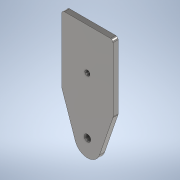
# Autodesk Inventor part: Frame2
Saved by Autodesk Inventor 2020 (Build 240168000, 168)
## iProperties
Created: 2022-06-23
Part Number: Frame2
Material: Steel, Carbon
Document SubType Name: Modeling
Designer: karimi2
Density: 7.85 g/cm^3
Appearance: Semi-Polished
Author: karimi2
Autodesk Inventor part; units mm, degrees
ref_plane "YZ Plane" through (0, 0, 0) normal (1, 0, 0) x (0, 1, 0)
ref_plane "XZ Plane" through (0, 0, 0) normal (0, 1, 0) x (-1, 0, 0)
ref_plane "XY Plane" through (0, 0, 0) normal (0, 0, 1) x (1, 0, 0)
sketch "Sketch1" plane through (0, 0, 0) normal (0, 0, 1) x (1, 0, 0)
  line L0 (0, 0) -> (0, 100) construction
  line L1 (0, 90) -> (-20, 90)
  line L2 (-20, 90) -> (-20, 37.5)
  arc A0 (-9.4595, 6.7568) -> (0, 0) centre (0, 10) ccw
  line L3 (-20, 37.5) -> (-9.4595, 6.7568)
  line L4 (0, 90) -> (20, 90)
  line L5 (20, 90) -> (20, 37.5)
  arc A1 (0, 0) -> (9.4595, 6.7568) centre (0, 10) ccw
  line L6 (20, 37.5) -> (9.4595, 6.7568)
  circle A2 centre (0, 57.5) radius 2
  circle A3 centre (0, 13.5) radius 2.6
  dimension "d0" = 100
  dimension "d1" = 20
  dimension "d2" = 90
  dimension "d3" = 52.5
  dimension "d4" = 10
  dimension "d5" = 20
  dimension "d6" = 32.5
  dimension "d7" = 4
  dimension "d8" = 24
  dimension "d9" = 5.2
  constraints: 14 end point, 5 point on line, 4 centre point, 4 point on circle, 3 symmetric about line, 2 vertical, 1 horizontal, 1 tangent, 1 other
  measures "d0" distance of L0.start L0.end
  measures "d1" distance of L1.start L1.end
  measures "d2" distance of L0.start L1.start
  measures "d3" distance of L1.end L2.end
  measures "d4" distance of L0.start A0.centre
  measures "d5" diameter of A0
  measures "d6" distance of L1.start A2.centre
  measures "d7" diameter of A2
  measures "d8" vertical distance of A3.centre L2.end
  measures "d9" diameter of A3
extrude "Extrusion1" add sketch "Sketch1" along normal mid plane 4
fillet "Fillet1" radius 2 4 edges at (20, 90, 0) (20, 37.5, 0) (-20, 37.5, 0) (-20, 90, 0)
body "Solid1"
